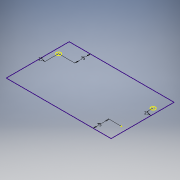
# Autodesk Inventor part: Estante01
Saved by Autodesk Inventor 2016 (Build 200138000, 138)
## iProperties
Created: 2018-06-25
Part Number: Estante01
Material: Wood (Birch)
Document SubType Name: Modeling
Designer: damia
Density: 0.55 g/cm^3
Appearance: Birch - Natural Polished
Mass: 2673 g
Surface Area: 5832 cm^2
Volume: 4860 cm^3
Author: damia
Autodesk Inventor part; units mm, degrees
ref_plane "YZ Plane" through (0, 0, 0) normal (1, 0, 0) x (0, 1, 0)
ref_plane "XZ Plane" through (0, 0, 0) normal (0, 1, 0) x (-1, 0, 0)
ref_plane "XY Plane" through (0, 0, 0) normal (0, 0, 1) x (1, 0, 0)
sketch "Sketch1" plane through (0, 0, 0) normal (0, 0, 1) x (1, 0, 0)
  circle A0 centre (-850, 150) radius 10.65 projected
  circle A1 centre (0, 150) radius 10.65 projected
  line L0 (-875, 225) -> (25, 225)
  line L1 (25, 225) -> (25, -75)
  line L2 (25, -75) -> (-875, -75)
  line L3 (-875, -75) -> (-875, 225)
  point P0 (0, 0)
  dimension "d0" = 75
  dimension "d1" = 25
  dimension "d2" = 25
  dimension "d3" = 75
  constraints: 8 end point, 2 parallel, 1 horizontal, 1 perpendicular
  measures "d0" distance from line of L0 A0.centre
  measures "d1" distance from line of L1 A1.centre
  measures "d2" distance from line of L3 A0.centre
  measures "d3" distance from line of point (0, 0) L2
extrude "Extrusion1" add sketch "Sketch1" along normal blind 18 contours A0 | A1 | L0 L1 L2 L3
body "Solid1"
